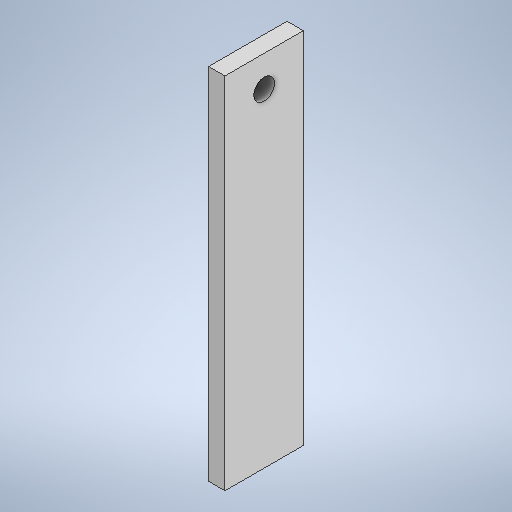
# Autodesk Inventor part: tallwall2
Saved by Autodesk Inventor 2025.1 (Build 291241000, 241)
## iProperties
Created: 2025-11-11
Part Number: tallwall2
Material: Generic
Document SubType Name: Modeling
Designer: mukund
Density: 1 g/cm^3
Appearance: Default
Author: mukund
Autodesk Inventor part; units mm, degrees
ref_plane "YZ Plane" through (0, 0, 0) normal (1, 0, 0) x (0, 1, 0)
ref_plane "XZ Plane" through (0, 0, 0) normal (0, 1, 0) x (-1, 0, 0)
ref_plane "XY Plane" through (0, 0, 0) normal (0, 0, 1) x (1, 0, 0)
sketch "Sketch1" plane through (0, 0, 0) normal (1, 0, 0) x (0, 1, 0)
  line L0 (0, 0) -> (220, 0)
  line L1 (220, 0) -> (220, -48)
  line L2 (220, -48) -> (0, -48)
  line L3 (0, -48) -> (0, 0)
  line L4 (0, -24) -> (201, -24)
  circle A0 centre (201, -24) radius 6.4
  dimension "d0" = 220
  dimension "d1" = 48
  dimension "d2" = 201
  dimension "d3" = 12.8
  constraints: 10 end point, 2 horizontal, 2 parallel, 1 centre point, 1 coincident, 1 midpoint, 1 perpendicular
  measures "d0" distance of L1.end L2.end
  measures "d1" distance of L0.end L1.end
  measures "d2" distance of L4.start L4.end
  measures "d3" diameter of A0
extrude "Extrusion1" add sketch "Sketch1" along normal blind 10
body "Solid1"
